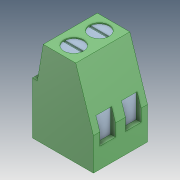
# Autodesk Inventor part: CAN_bus_wire
Saved by Autodesk Inventor 2020 (Build 240168000, 168)
## iProperties
Created: 2020-09-27
Part Number: CAN_bus_wire
Material: Generic
Document SubType Name: Modeling
Designer: DELL
Density: 1 g/cm^3
Appearance: Smooth - Dark Forest Green
Author: DELL
Autodesk Inventor part; units mm, degrees
ref_plane "YZ Plane" through (0, 0, 0) normal (1, 0, 0) x (0, 1, 0)
ref_plane "XZ Plane" through (0, 0, 0) normal (0, 1, 0) x (-1, 0, 0)
sketch "Sketch1" plane through (0, 0, 0) normal (0, 0, 1) x (1, 0, 0)
  line L0 (0, 0) -> (0, 3.3)
  line L1 (0, 3.3) -> (-1.8, 8.8)
  line L2 (-1.8, 8.8) -> (-5.1, 8.8)
  line L3 (-5.1, 8.8) -> (-5.7, 5.3)
  line L4 (-5.7, 5.3) -> (-6.2, 5.3)
  line L5 (-6.2, 5.3) -> (-6.2, 0)
  line L6 (-6.2, 0) -> (0, 0)
  dimension "d0" = 3.3
  dimension "d1" = 3.3
  dimension "d2" = 8.8
  dimension "d3" = 1.8
  dimension "d4" = 5.3
  dimension "d5" = 6.2
  dimension "d6" = 0.5
  constraints: 14 end point, 3 perpendicular, 1 parallel, 1 vertical
  measures "d0" distance of L0.start L0.end
  measures "d1" distance of L1.end L2.end
  measures "d2" distance between parallel lines of L6 L2
  measures "d3" distance from line of L1.end L0
  measures "d4" distance of L4.end L5.end
  measures "d5" distance between parallel lines of L0 L5
  measures "d6" distance of L3.end L4.end
extrude "Extrusion1" add sketch "Sketch1" along normal blind 5.5
ref_plane "Work Plane2" through (0, 0, 4.02) normal (0, 0, 1) x (1, 0, 0)
ref_plane "Work Plane1" through (0, 0, 2.75) normal (0, 0, 1) x (1, 0, 0)
sketch "Sketch3" plane through (0, 0, 4.02) normal (0, 0, 1) x (1, 0, 0)
  line L0 (-6.2, 5.3) -> (-6.2, 0) projected
  line L1 (-6.2, 5.1) -> (-5.2, 4.1)
  line L2 (-5.2, 4.1) -> (-2.3, 4.1)
  line L3 (-2.3, 4.1) -> (-2.3, 1.2)
  line L4 (-2.3, 1.2) -> (-5.2, 1.2)
  line L5 (-5.2, 1.2) -> (-6.2, 0.2)
  line L6 (-6.2, 5.1) -> (-6.2, 0.2)
  line L7 (-5.7, 5.3) -> (-6.2, 5.3) projected
  line L8 (-6.2, 0) -> (0, 0) projected
  line L9 (-6.2, 2.65) -> (0, 2.65) construction
  line L10 (0, 0) -> (0, 3.3) construction
  dimension "d10" = 0.2
  dimension "d11" = 0.2
  dimension "d12" = 1
  dimension "d13" = 1
  constraints: 14 end point, 4 point on line, 2 horizontal, 1 collinear, 1 midpoint, 1 perpendicular, 1 vertical, 2 other
  measures "d10" distance from line of L7 L1.start
  measures "d11" distance from line of L8 L5.end
  measures "d12" distance from line of L0 L1.end
  measures "d13" horizontal distance of L1.start L1.end
extrude "Extrusion2" cut sketch "Sketch3" along normal mid plane 2.3
mirror "Mirror1" about plane through (0, 0, 2.75) normal (0, 0, 1) of "Extrusion2"
sketch "Sketch4" plane through (0, 0, 0) normal (1, 0, 0) x (0, 0, -1)
  line L0 (-4.85, 4.55) -> (-3.25, 4.55)
  line L1 (-3.25, 4.55) -> (-3.25, 2.05)
  line L2 (-3.25, 2.05) -> (-4.85, 2.05)
  line L3 (-4.85, 2.05) -> (-4.85, 4.55)
  line L4 (-4.85, 4.55) -> (-3.25, 2.05) construction
  line L5 (-3.25, 4.55) -> (-4.85, 2.05) construction
  line L6 (-2.25, 4.55) -> (-0.65, 4.55)
  line L7 (-0.65, 4.55) -> (-0.65, 2.05)
  line L8 (-0.65, 2.05) -> (-2.25, 2.05)
  line L9 (-2.25, 2.05) -> (-2.25, 4.55)
  line L10 (-2.25, 4.55) -> (-0.65, 2.05) construction
  line L11 (-0.65, 4.55) -> (-2.25, 2.05) construction
  line L12 (0, 8.8) -> (-5.5, 8.8) construction
  line L13 (-2.75, 8.8) -> (-2.75, 0) construction
  line L14 (0, 0) -> (-5.5, 0) construction
  line L15 (0, 3.3) -> (-5.5, 3.3) construction
  point P0 (-4.05, 3.3)
  point P1 (-1.45, 3.3)
  dimension "d16" = 1.6
  dimension "d17" = 2.5
  dimension "d18" = 1
  constraints: 26 end point, 6 midpoint, 4 parallel, 2 collinear, 2 horizontal, 2 perpendicular, 1 point on line, 3 other
  measures "d16" distance of L0.start L0.end
  measures "d17" distance of L2.end L0.start
  measures "d18" distance between parallel lines of L9 L1
extrude "Extrusion3" cut sketch "Sketch4" against normal blind 0.5
sketch "Sketch5" plane through (-5.1, 8.8, 0) normal (0, 1, 0) x (1, 0, 0)
  circle A0 centre (1.65, -4.05) radius 1
  line L0 (-1.1, -5.5) -> (5.1, -5.5) construction
  line L1 (3.3, 0) -> (3.3, -5.5) construction
  line L2 (0, -5.5) -> (3.3, -5.5) construction
  line L3 (3.3, -5.5) -> (3.3, 0) construction
  line L4 (3.3, 0) -> (0, 0) construction
  line L5 (0, 0) -> (0, -5.5) construction
  line L6 (1.65, -5.5) -> (1.65, 0) construction
  line L7 (0, 0) -> (0, -5.5) construction
  line L8 (0, -2.75) -> (3.3, -2.75) construction
  line L9 (0.655, -4.15) -> (2.645, -4.15)
  line L10 (2.645, -3.95) -> (0.655, -3.95)
  circle A1 centre (1.65, -1.45) radius 1
  line L11 (1.65, 0) -> (1.65, -5.5) construction
  line L12 (0.655, -1.35) -> (2.645, -1.35)
  line L13 (2.645, -1.55) -> (0.655, -1.55)
  point P0 (5.1, 0)
  dimension "d21" = 2
  dimension "d22" = 0.2
  dimension "d23" = 1.3
  dimension "d24" = 0.1
  constraints: 22 end point, 8 point on circle, 7 symmetric about line, 4 midpoint, 4 point on line, 3 horizontal, 2 centre point, 2 parallel, 1 perpendicular, 1 other
  measures "d21" diameter of A0
  measures "d22" distance between parallel lines of L10 L9
  measures "d23" distance from line of L8 A0.centre
  measures "d24" distance from line of A0.centre L10
extrude "Extrusion4" cut sketch "Sketch5" against normal blind 0.1 contours L10 A0 | A0 L9 | L12 A1 | A1 L13
extrude "Extrusion5" cut sketch "Sketch5" against normal blind 0.2 contours A0 L9 L10 | A1 L13 L12
sketch "Sketch6" plane through (-6.2, 0, 0) normal (0, -1, 0) x (1, 0, 0)
  circle A0 centre (3.1, 4.02) radius 0.35
  circle A1 centre (3.1, 1.48) radius 0.35
  line L0 (6.2, 2.25) -> (6.2, 3.25) construction
  line L1 (6.2, 2.75) -> (0, 2.75) construction
  line L2 (0, 2.63) -> (1, 2.63) construction
  line L3 (6.2, 0) -> (6.2, 5.5) construction
  dimension "d29" = 0.7
  dimension "d30" = 2.54
  dimension "d31" = 3.1
  constraints: 2 centre point, 2 end point, 1 equal radius, 1 midpoint, 1 parallel, 1 symmetric about line
  measures "d29" diameter of A0
  measures "d30" distance of A1.centre A0.centre
  measures "d31" distance from line of L3 A0.centre
extrude "Extrusion6" cut sketch "Sketch6" against normal blind 0.2
body "Solid1"
